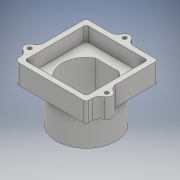
# Autodesk Inventor part: MS_FocusSliderv11
Saved by Autodesk Inventor 2017 (Build 210142000, 142)
## iProperties
Created: 2017-12-13
Part Number: MS_FocusSliderv11
Material: Generic
Document SubType Name: Modeling
Designer: andrew
Density: 1 g/cm^3
Appearance: Default
Author: andrew
Autodesk Inventor part; units mm, degrees
ref_plane "YZ Plane" through (0, 0, 0) normal (1, 0, 0) x (0, 1, 0)
ref_plane "XZ Plane" through (0, 0, 0) normal (0, 1, 0) x (-1, 0, 0)
ref_plane "XY Plane" through (0, 0, 0) normal (0, 0, 1) x (1, 0, 0)
sketch "Sketch1" plane through (0, 0, 0) normal (0, 0, 1) x (1, 0, 0)
  circle A0 centre (0, 0) radius 5.75
  line L0 (2.2382, 4.0759) -> (-2.2382, 4.0759)
  arc A1 (-2.2382, 4.0759) -> (2.2382, 4.0759) centre (0, 0) ccw
  dimension "d0" = 11.5
  dimension "d50" = 9.3
  constraints: 2 centre point, 2 end point, 2 point on circle, 1 coincident
  measures "d0" diameter of A0
  measures "d50" diameter of A1
extrude "Extrusion1" add sketch "Sketch1" along normal blind 7
sketch "Sketch2" plane through (0, 0, 0) normal (0, 0, -1) x (-1, 0, 0)
  line L0 (-1.25, 5.125) -> (1.25, 5.125) construction
  circle A0 centre (0, 0) radius 5.75 construction
  line L1 (0, 0) -> (0, 9.5083) construction
  circle A1 centre (0, 0) radius 5.75 construction
  line L2 (0, 5.75) -> (0, 7.7304) construction
  line L3 (0, 5.125) -> (0, 7.5987) construction
  line L4 (-1.25, 5.125) -> (-1.25, 6.125) construction
  line L5 (-1.25, 6.125) -> (1.25, 6.125)
  line L6 (1.25, 6.125) -> (1.25, 4.5986)
  line L7 (1.25, 4.5986) -> (-1.25, 4.5986)
  line L8 (-1.25, 4.5986) -> (-1.25, 6.125)
  dimension "d3" = 2.5
  dimension "d4" = 1
  constraints: 18 end point, 3 vertical, 2 horizontal, 2 parallel, 2 point on line, 1 midpoint, 1 perpendicular, 1 vertical alignment, 1 other
  measures "d3" distance of L0.start L0.end
  measures "d4" distance of L0.start L4.end
extrude "Extrusion2" add sketch "Sketch2" against normal blind 5
sketch "Sketch3" plane through (0, 0, 7) normal (0, 0, 1) x (1, 0, 0)
  line L0 (6.5, -7) -> (-6, -7)
  arc A0 (-7, -6) -> (-6, -7) centre (-6, -6) ccw
  arc A1 (-6.5, 7) -> (-7, 6.5) centre (-6.5, 6.5) ccw
  arc A2 (7, 6.5) -> (6.5, 7) centre (6.5, 6.5) ccw
  arc A3 (6.5, -7) -> (7, -6.5) centre (6.5, -6.5) ccw
  line L1 (-5.5, -6) -> (5.5, -6)
  line L2 (6, -5.5) -> (6, 5.5)
  line L3 (5.5, 6) -> (-5.5, 6)
  line L4 (-6, 5.5) -> (-6, -5.5)
  arc A4 (-6, -5.5) -> (-5.5, -6) centre (-5.5, -5.5) ccw
  arc A5 (5.5, -6) -> (6, -5.5) centre (5.5, -5.5) ccw
  arc A6 (6, 5.5) -> (5.5, 6) centre (5.5, 5.5) ccw
  arc A7 (-5.5, 6) -> (-6, 5.5) centre (-5.5, 5.5) ccw
  line L5 (-10.9736, -8.9739) -> (-4.3472, -8.9739) construction
  arc A8 (-7.9, -2.5835) -> (-7.9, -4.4165) centre (-7.5, -3.5) ccw
  circle A9 centre (-7.5, -3.5) radius 0.375
  arc A10 (0.9165, 7.9) -> (-0.9165, 7.9) centre (0, 7.5) ccw
  circle A11 centre (0, 7.5) radius 0.375
  arc A12 (7.9, -4.4165) -> (7.9, -2.5835) centre (7.5, -3.5) ccw
  circle A13 centre (7.5, -3.5) radius 0.375
  line L6 (-7, -6) -> (-7, -5.7913)
  line L7 (-7, -1.2087) -> (-7, 6.5)
  arc A14 (-7, -5.7913) -> (-7.9, -4.4165) centre (-8.5, -5.7913) ccw
  arc A15 (-7.9, -2.5835) -> (-7, -1.2087) centre (-8.5, -1.2087) ccw
  line L8 (-6.5, 7) -> (-2.2913, 7)
  line L9 (2.2913, 7) -> (6.5, 7)
  arc A16 (-2.2913, 7) -> (-0.9165, 7.9) centre (-2.2913, 8.5) ccw
  arc A17 (0.9165, 7.9) -> (2.2913, 7) centre (2.2913, 8.5) ccw
  line L10 (7, 6.5) -> (7, -1.2087)
  line L11 (7, -5.7913) -> (7, -6.5)
  arc A18 (7.9, -4.4165) -> (7, -5.7913) centre (8.5, -5.7913) ccw
  arc A19 (7, -1.2087) -> (7.9, -2.5835) centre (8.5, -1.2087) ccw
  line L12 (-2.2382, 4.0759) -> (2.2382, 4.0759) projected
  arc A20 (-2.2382, 4.0759) -> (2.2382, 4.0759) centre (0, 0) ccw projected
  point P0 (7, 7)
  point P1 (-7, 7)
  point P2 (7, -7)
  point P3 (-7, -4.366)
  point P4 (-7, -2.634)
  point P5 (-0.866, 7)
  point P6 (0.866, 7)
  point P7 (7, -2.634)
  point P8 (7, -4.366)
  dimension "d9" = 14
  dimension "d11" = 1
  dimension "d13" = 1
  dimension "d14" = 0.5
  dimension "d15" = 2
  dimension "d16" = 0.75
  dimension "d18" = 0.75
  dimension "d19" = 2
  dimension "d20" = 0.75
  dimension "d21" = 1.5
  dimension "d22" = 1.5
  dimension "d23" = 1.5
  constraints: 40 point on circle, 34 tangent, 24 end point, 20 centre point, 8 equal radius, 8 parallel, 7 point on line, 6 coincident, 5 perpendicular
  measures "d9" distance of point (7, 7) point (7, -7)
  measures "d11" radius of A0
  measures "d13" distance between parallel lines of L0 L1
  measures "d14" radius of A4
  measures "d15" diameter of A8
  measures "d16" diameter of A9
  measures "d18" diameter of A11
  measures "d19" diameter of A12
  measures "d20" diameter of A13
  measures "d21" radius of A14
  measures "d22" radius of A16
  measures "d23" radius of A18
extrude "Extrusion3" add sketch "Sketch3" along normal blind 1 contours L0 A0 L6 A14 A8 A15 L7 A1 L8 A16 A10 A17 L9 A2 L10 A19 A12 A18 L11 A3 | A4 L4 A7 L3 A6 L2 A5 L1
sketch "Sketch4" plane through (0, 0, 8) normal (0, 0, 1) x (1, 0, 0)
  line L0 (6.5, -7) -> (-6, -7)
  arc A0 (-7, -6) -> (-6, -7) centre (-6, -6) ccw
  arc A1 (-6.5, 7) -> (-7, 6.5) centre (-6.5, 6.5) ccw
  arc A2 (7, 6.5) -> (6.5, 7) centre (6.5, 6.5) ccw
  arc A3 (6.5, -7) -> (7, -6.5) centre (6.5, -6.5) ccw
  line L1 (-5.5, -6) -> (5.5, -6)
  line L2 (6, -5.5) -> (6, 5.5)
  line L3 (5.5, 6) -> (-5.5, 6)
  line L4 (-6, 5.5) -> (-6, -5.5)
  arc A4 (-6, -5.5) -> (-5.5, -6) centre (-5.5, -5.5) ccw
  arc A5 (5.5, -6) -> (6, -5.5) centre (5.5, -5.5) ccw
  arc A6 (6, 5.5) -> (5.5, 6) centre (5.5, 5.5) ccw
  arc A7 (-5.5, 6) -> (-6, 5.5) centre (-5.5, 5.5) ccw
  line L5 (-10.9736, -8.9739) -> (-4.3472, -8.9739) construction
  arc A8 (-7.9, -2.5835) -> (-7.9, -4.4165) centre (-7.5, -3.5) ccw
  circle A9 centre (-7.5, -3.5) radius 0.375
  arc A10 (0.9165, 7.9) -> (-0.9165, 7.9) centre (0, 7.5) ccw
  circle A11 centre (0, 7.5) radius 0.375
  arc A12 (7.9, -4.4165) -> (7.9, -2.5835) centre (7.5, -3.5) ccw
  circle A13 centre (7.5, -3.5) radius 0.375
  line L6 (-7, -6) -> (-7, -5.7913)
  line L7 (-7, -1.2087) -> (-7, 6.5)
  arc A14 (-7, -5.7913) -> (-7.9, -4.4165) centre (-8.5, -5.7913) ccw
  arc A15 (-7.9, -2.5835) -> (-7, -1.2087) centre (-8.5, -1.2087) ccw
  line L8 (-6.5, 7) -> (-2.2913, 7)
  line L9 (2.2913, 7) -> (6.5, 7)
  arc A16 (-2.2913, 7) -> (-0.9165, 7.9) centre (-2.2913, 8.5) ccw
  arc A17 (0.9165, 7.9) -> (2.2913, 7) centre (2.2913, 8.5) ccw
  line L10 (7, 6.5) -> (7, -1.2087)
  line L11 (7, -5.7913) -> (7, -6.5)
  arc A18 (7.9, -4.4165) -> (7, -5.7913) centre (8.5, -5.7913) ccw
  arc A19 (7, -1.2087) -> (7.9, -2.5835) centre (8.5, -1.2087) ccw
  arc A20 (4.3875, 1) -> (4.3875, -1) centre (0, 0) ccw
  circle A21 centre (0, 0) radius 4.5
  point P0 (7, 7)
  point P1 (-7, 7)
  point P2 (7, -7)
  point P3 (-7, -4.366)
  point P4 (-7, -2.634)
  point P5 (-0.866, 7)
  point P6 (0.866, 7)
  point P7 (7, -2.634)
  point P8 (7, -4.366)
  dimension "d26" = 14
  dimension "d27" = 1
  dimension "d28" = 1
  dimension "d29" = 0.5
  dimension "d30" = 2
  dimension "d31" = 0.75
  dimension "d32" = 0.75
  dimension "d33" = 2
  dimension "d34" = 0.75
  dimension "d35" = 1.5
  dimension "d36" = 1.5
  dimension "d37" = 1.5
  constraints: 42 point on circle, 34 tangent, 24 end point, 22 centre point, 9 equal radius, 8 parallel, 7 coincident, 7 point on line, 5 perpendicular
  measures "d26" distance of point (7, 7) point (7, -7)
  measures "d27" radius of A0
  measures "d28" distance between parallel lines of L0 L1
  measures "d29" radius of A4
  measures "d30" diameter of A8
  measures "d31" diameter of A9
  measures "d32" diameter of A11
  measures "d33" diameter of A12
  measures "d34" diameter of A13
  measures "d35" radius of A14
  measures "d36" radius of A16
  measures "d37" radius of A18
extrude "Extrusion4" add sketch "Sketch4" along normal blind 2.8 contours L0 A0 L6 A14 A8 A15 L7 A1 L8 A16 A10 A17 L9 A2 L10 A19 A12 A18 L11 A3
sketch "Sketch5" plane through (-1.25, 6.125, 0) normal (0, 1, 0) x (1, 0, 0)
  line L0 (1.8283, -3.8925) -> (1.8437, -3.7979)
  line L1 (0.8374, -4.1796) -> (0.9116, -4.2402)
  line L2 (0.7226, -3.4732) -> (0.7738, -3.3922)
  line L3 (1.7534, -0.9317) -> (1.798, -1.0165)
  line L4 (0.8374, -1.6796) -> (0.9116, -1.7402)
  line L5 (0.7738, -0.8922) -> (0.8374, -0.8204)
  line L6 (0, 0) -> (2.5, 0)
  line L7 (0, 0) -> (0, -5)
  circle A0 centre (1.25, -1.25) radius 0.5937
  circle A1 centre (1.25, -3.75) radius 0.5937
  point P0 (1.25, 0)
  point P1 (1.0843, -1.8221)
  dimension "d40" = 1.1874
  constraints: 16 end point, 6 tangent, 2 centre point
  measures "d40" diameter of A1
extrude "Extrusion5" cut sketch "Sketch5" against normal blind 5
fillet "Fillet1" radius 2 2 edges at (-1.25, 5.6125, 2.5) (1.25, 5.6125, 2.5)
chamfer "Chamfer1" distance 0.5 angle 45 1 edges at (0, 4.0759, 0)
body "Solid1"
